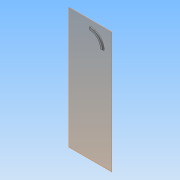
# Autodesk Inventor part: HOT ThermoTop x2
Saved by Autodesk Inventor 2013 (Build 170138000, 138)
## iProperties
Created: 2018-07-29
Part Number: HOT ThermoTop x2
Material: Rubber, Butyl
Document SubType Name: Modeling
Designer: Jeff Vyduna
Density: 1 g/cm^3
Author: Jeff Vyduna
Autodesk Inventor part; units mm, degrees
ref_plane "YZ Plane" through (0, 0, 0) normal (1, 0, 0) x (0, 1, 0)
ref_plane "XZ Plane" through (0, 0, 0) normal (0, 1, 0) x (-1, 0, 0)
ref_plane "XY Plane" through (0, 0, 0) normal (0, 0, 1) x (1, 0, 0)
ref_plane "Work Plane1" through (0, 0, 0) normal (0, 0, 1) x (1, 0, 0)
sketch "Sketch1" plane through (0, 0, 0) normal (0, 0, 1) x (1, 0, 0)
  line L0 (156.7398, 908.0528) -> (93.2398, 908.0528) projected
  line L1 (-389.3602, 908.0528) -> (-452.8602, 908.0528) projected
  arc A0 (156.7398, 908.0528) -> (-452.8602, 908.0528) centre (-148.0602, 908.0528) ccw projected
  arc A1 (93.2398, 908.0528) -> (-148.0602, 1149.3528) centre (-148.0602, 908.0528) ccw
  arc A2 (156.7398, 908.0528) -> (-148.0602, 1212.8528) centre (-148.0602, 908.0528) ccw
  line L2 (93.2398, 908.0528) -> (156.7398, 908.0528)
  line L3 (-148.0602, 1212.8528) -> (-148.0602, 1149.3528)
  point P0 (0, 0)
  dimension "d0" = 304.8
  constraints: 4 end point, 4 point on circle, 3 concentric, 2 centre point, 1 vertical
  measures "d0" horizontal distance of L0.start L3.start
extrude "Extrusion1" add sketch "Sketch1" along normal blind 18.034
sketch "Sketch2" plane through (0, 0, 18.034) normal (0, 0, 1) x (1, 0, 0)
  arc A0 (156.7398, 908.0528) -> (-148.0602, 1212.8528) centre (-148.0602, 908.0528) ccw projected
  arc A1 (144.0398, 908.0528) -> (-148.0602, 1200.1528) centre (-148.0602, 908.0528) ccw
  arc A2 (131.8478, 908.0528) -> (-148.0602, 1187.9608) centre (-148.0602, 908.0528) ccw
  line L0 (156.7398, 908.0528) -> (93.2398, 908.0528) projected
  line L1 (93.2398, 908.0528) -> (156.7398, 908.0528) projected
  arc A3 (-148.0602, 1200.1528) -> (-148.0602, 1187.9608) centre (-148.0069, 1194.0568) ccw
  line L2 (-148.0602, 1212.8528) -> (-148.0602, 1149.3528) projected
  arc A4 (131.8478, 908.0528) -> (144.0398, 908.0528) centre (137.9438, 908.0528) ccw
  point P0 (0, 0)
  point P1 (-154.1031, 1194.0568)
  dimension "d3" = 12.7
  dimension "pathW" = 12.192
  constraints: 9 point on circle, 4 centre point, 4 point on line, 2 concentric, 2 line through centre, 2 tangent, 1 horizontal alignment
  measures "d3" distance of A1.start L0.start
  measures "pathW" radial gap between concentric circles of A1 A2
extrude "Extrusion2" cut sketch "Sketch2" against normal blind 12.7 contours L0 A2 L2 A1
body "Solid1"
